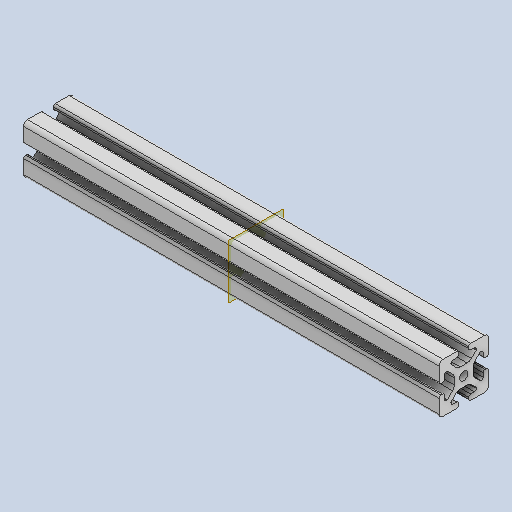
# Autodesk Inventor part: \
Saved by Autodesk Inventor 2025.2 (Build 292293000, 293)
## iProperties
Created: 2026-02-05
Part Number: \
Material: Generic
Document SubType Name: Modeling
Designer: composite
Density: 1 g/cm^3
Appearance: Default
Author: composite
Autodesk Inventor part; units mm, degrees
ref_plane "YZ Plane" through (0, 0, 0) normal (1, 0, 0) x (0, 1, 0)
ref_plane "XZ Plane" through (0, 0, 0) normal (0, 1, 0) x (-1, 0, 0)
ref_plane "XY Plane" through (0, 0, 0) normal (0, 0, 1) x (1, 0, 0)
derived "4040_REPRESENTATIVE.ipt"
sketch "Sketch2" plane through (20, -17.0184, 40) normal (1, 0, 0) x (0, 0, -1)
  arc A0 (15.94, -0.0762) -> (14.37, 1.4938) centre (14.37, -0.0762) ccw projected
  line L0 (14.37, 1.4938) -> (11.285, 1.4938) projected
  arc A1 (9.715, 3.0638) -> (11.285, 1.4938) centre (11.285, 3.0638) ccw projected
  line L1 (9.715, 3.0638) -> (9.715, 3.5259) projected
  arc A2 (9.9376, 4.0633) -> (9.715, 3.5259) centre (10.475, 3.5259) ccw projected
  line L2 (9.9376, 4.0633) -> (13.7829, 7.9086) projected
  arc A3 (17.2227, 9.3334) -> (13.7829, 7.9086) centre (17.2227, 4.4688) ccw projected
  line L3 (17.2227, 9.3334) -> (22.7773, 9.3334) projected
  arc A4 (26.2171, 7.9086) -> (22.7773, 9.3334) centre (22.7773, 4.4688) ccw projected
  line L4 (26.2171, 7.9086) -> (30.0624, 4.0633) projected
  arc A5 (30.285, 3.5259) -> (30.0624, 4.0633) centre (29.525, 3.5259) ccw projected
  line L5 (30.285, 3.5259) -> (30.285, 3.0638) projected
  arc A6 (28.715, 1.4938) -> (30.285, 3.0638) centre (28.715, 3.0638) ccw projected
  line L6 (28.715, 1.4938) -> (25.63, 1.4938) projected
  arc A7 (25.63, 1.4938) -> (24.06, -0.0762) centre (25.63, -0.0762) ccw projected
  line L7 (24.06, -0.0762) -> (24.06, -1.4116) projected
  arc A8 (24.06, -1.4116) -> (25.63, -2.9816) centre (25.63, -1.4116) ccw projected
  line L8 (25.63, -2.9816) -> (36.83, -2.9816) projected
  arc A9 (36.83, -2.9816) -> (40, 0.1884) centre (36.83, 0.1884) ccw projected
  line L9 (40, 0.1884) -> (40, 11.3884) projected
  arc A10 (40, 11.3884) -> (38.43, 12.9584) centre (38.43, 11.3884) ccw projected
  line L10 (38.43, 12.9584) -> (37.25, 12.9584) projected
  arc A11 (37.25, 12.9584) -> (35.68, 11.3884) centre (37.25, 11.3884) ccw projected
  line L11 (35.68, 11.3884) -> (35.68, 8.303) projected
  arc A12 (34.11, 6.733) -> (35.68, 8.303) centre (34.11, 8.303) ccw projected
  line L12 (34.11, 6.733) -> (33.6201, 6.733) projected
  arc A13 (33.1637, 7.0714) -> (33.6201, 6.733) centre (33.8117, 7.4684) ccw projected
  line L13 (33.1637, 7.0714) -> (29.0762, 11.1588) projected
  arc A14 (27.685, 14.5176) -> (29.0762, 11.1588) centre (32.435, 14.5176) ccw projected
  line L14 (27.685, 14.5176) -> (27.685, 19.5192) projected
  arc A15 (29.0762, 22.8779) -> (27.685, 19.5192) centre (32.435, 19.5192) ccw projected
  line L15 (29.0762, 22.8779) -> (33.2795, 27.0812) projected
  arc A16 (33.8169, 27.3038) -> (33.2795, 27.0812) centre (33.8169, 26.5438) ccw projected
  line L16 (33.8169, 27.3038) -> (34.11, 27.3038) projected
  arc A17 (35.68, 25.7338) -> (34.11, 27.3038) centre (34.11, 25.7338) ccw projected
  line L17 (35.68, 25.7338) -> (35.68, 22.6484) projected
  arc A18 (35.68, 22.6484) -> (37.25, 21.0784) centre (37.25, 22.6484) ccw projected
  line L18 (37.25, 21.0784) -> (38.43, 21.0784) projected
  arc A19 (38.43, 21.0784) -> (40, 22.6484) centre (38.43, 22.6484) ccw projected
  line L19 (40, 22.6484) -> (40, 33.8484) projected
  arc A20 (40, 33.8484) -> (36.83, 37.0184) centre (36.83, 33.8484) ccw projected
  line L20 (36.83, 37.0184) -> (25.63, 37.0184) projected
  arc A21 (25.63, 37.0184) -> (24.06, 35.4484) centre (25.63, 35.4484) ccw projected
  line L21 (24.06, 35.4484) -> (24.06, 34.113) projected
  arc A22 (24.06, 34.113) -> (25.63, 32.543) centre (25.63, 34.113) ccw projected
  line L22 (25.63, 32.543) -> (28.715, 32.543) projected
  arc A23 (30.285, 30.973) -> (28.715, 32.543) centre (28.715, 30.973) ccw projected
  line L23 (30.285, 30.973) -> (30.285, 30.5109) projected
  arc A24 (30.0624, 29.9735) -> (30.285, 30.5109) centre (29.525, 30.5109) ccw projected
  line L24 (30.0624, 29.9735) -> (26.2171, 26.1282) projected
  arc A25 (22.7773, 24.7034) -> (26.2171, 26.1282) centre (22.7773, 29.5679) ccw projected
  line L25 (22.7773, 24.7034) -> (17.2227, 24.7034) projected
  arc A26 (13.7829, 26.1282) -> (17.2227, 24.7034) centre (17.2227, 29.5679) ccw projected
  line L26 (13.7829, 26.1282) -> (9.9376, 29.9735) projected
  arc A27 (9.715, 30.5109) -> (9.9376, 29.9735) centre (10.475, 30.5109) ccw projected
  line L27 (9.715, 30.5109) -> (9.715, 30.973) projected
  arc A28 (11.285, 32.543) -> (9.715, 30.973) centre (11.285, 30.973) ccw projected
  line L28 (11.285, 32.543) -> (14.37, 32.543) projected
  arc A29 (14.37, 32.543) -> (15.94, 34.113) centre (14.37, 34.113) ccw projected
  line L29 (15.94, 34.113) -> (15.94, 35.4484) projected
  arc A30 (15.94, 35.4484) -> (14.37, 37.0184) centre (14.37, 35.4484) ccw projected
  line L30 (14.37, 37.0184) -> (3.17, 37.0184) projected
  arc A31 (3.17, 37.0184) -> (0, 33.8484) centre (3.17, 33.8484) ccw projected
  line L31 (0, 33.8484) -> (0, 22.5913) projected
  arc A32 (0, 22.5913) -> (1.57, 21.0213) centre (1.57, 22.5913) ccw projected
  line L32 (1.57, 21.0213) -> (2.75, 21.0213) projected
  arc A33 (2.75, 21.0213) -> (4.32, 22.5913) centre (2.75, 22.5913) ccw projected
  line L33 (4.32, 22.5913) -> (4.32, 25.494) projected
  arc A34 (5.9448, 27.0631) -> (4.32, 25.494) centre (5.89, 25.494) ccw projected
  line L34 (5.9448, 27.0631) -> (6.2801, 27.0514) projected
  arc A35 (6.9595, 26.8422) -> (6.2801, 27.0514) centre (6.4221, 26.3048) ccw projected
  line L35 (6.9595, 26.8422) -> (10.9238, 22.8779) projected
  arc A36 (12.315, 19.5192) -> (10.9238, 22.8779) centre (7.565, 19.5192) ccw projected
  line L36 (12.315, 19.5192) -> (12.315, 14.5176) projected
  arc A37 (10.9238, 11.1588) -> (12.315, 14.5176) centre (7.565, 14.5176) ccw projected
  line L37 (10.9238, 11.1588) -> (6.7205, 6.9556) projected
  arc A38 (6.1831, 6.733) -> (6.7205, 6.9556) centre (6.1831, 7.493) ccw projected
  line L38 (6.1831, 6.733) -> (5.89, 6.733) projected
  arc A39 (4.32, 8.303) -> (5.89, 6.733) centre (5.89, 8.303) ccw projected
  line L39 (4.32, 8.303) -> (4.32, 11.2604) projected
  arc A40 (4.32, 11.2604) -> (2.75, 12.8979) centre (2.7515, 11.3279) ccw projected
  line L40 (2.75, 12.8979) -> (1.57, 12.8979) projected
  arc A41 (1.57, 12.8979) -> (0, 11.2604) centre (1.5685, 11.3279) ccw projected
  line L41 (0, 11.2604) -> (0, 0) projected
  arc A42 (0, 0) -> (3.3254, -2.9816) centre (3.1646, 0.1843) ccw projected
  line L42 (3.3254, -2.9816) -> (14.37, -2.9816) projected
  arc A43 (14.37, -2.9816) -> (15.94, -1.4116) centre (14.37, -1.4116) ccw projected
  line L43 (15.94, -1.4116) -> (15.94, -0.0762) projected
  circle A44 centre (20, 17.0184) radius 3.4 projected
  point P0 (40, 17.0184)
extrude "Extrusion1" add sketch "Sketch2" along normal blind 336.5
ref_plane "Work Plane1" through (188.25, -17.0184, 40) normal (1, 0, 0) x (0, 0, -1)
ref_plane "Work Plane2" through (188.25, -17.0184, 40) normal (-1, 0, 0) x (0, 0, 1)
body "Solid1"
